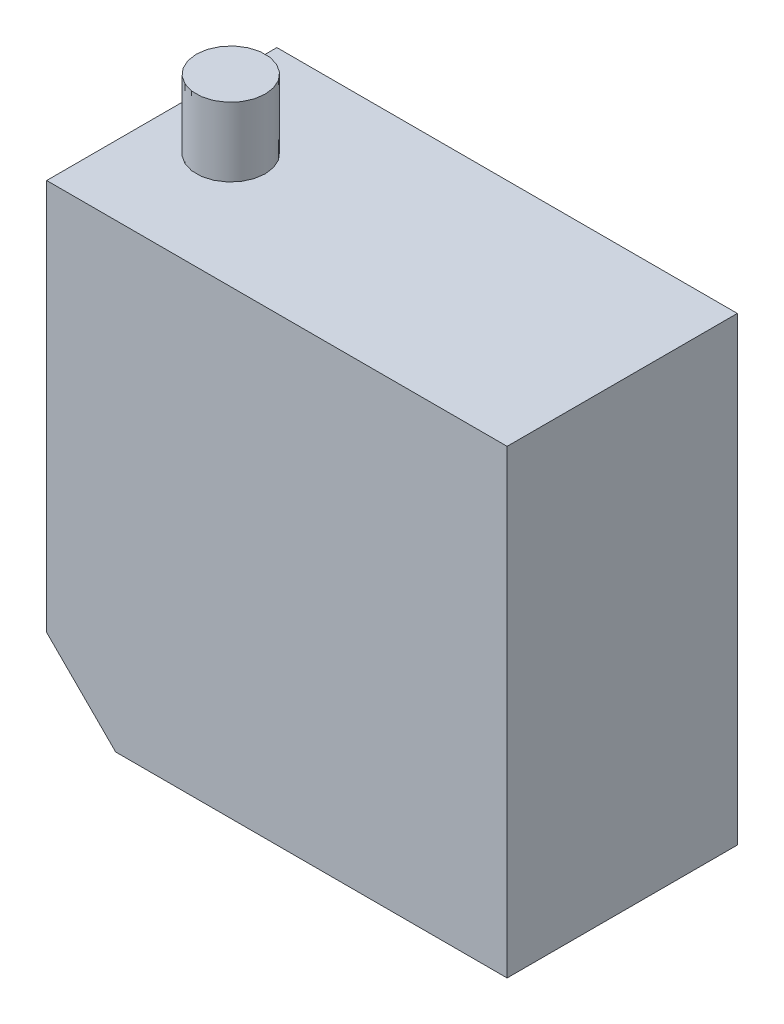
# Autodesk Inventor part: Finger Servo
Saved by Autodesk Inventor 2023 (Build 270158000, 158)
## iProperties
Created: 2023-09-27
Part Number: Finger Servo
Material: Generic
Document SubType Name: Modeling
Designer: Turnt
Density: 1 g/cm^3
Appearance: Default
Author: Turnt
Autodesk Inventor part; units mm, degrees
ref_plane "YZ Plane" through (0, 0, 0) normal (1, 0, 0) x (0, 1, 0)
ref_plane "XZ Plane" through (0, 0, 0) normal (0, 1, 0) x (-1, 0, 0)
ref_plane "XY Plane" through (0, 0, 0) normal (0, 0, 1) x (1, 0, 0)
sketch "Sketch1" plane through (0, 0, 0) normal (0, 0, 1) x (1, 0, 0)
  line L0 (3.8073, 0) -> (25.4, 0)
  line L1 (25.4, 0) -> (25.4, 25.4)
  line L2 (25.4, 25.4) -> (0, 25.4)
  line L3 (0, 25.4) -> (0, 3.8073)
  line L4 (0, 3.8073) -> (3.8073, 0)
  line L5 (0, 3.8073) -> (5.3843, 3.8073) construction
  point P0 (0, 0)
  dimension "d2" = 25.4
  dimension "d3" = 25.4
  dimension "d4" = 45
  constraints: 12 end point, 2 horizontal, 2 parallel, 1 equal length, 1 perpendicular
  measures "d2" distance of L2.end L1.end
  measures "d3" distance of L1.end L0.end
  measures "d4" angle of L4 L5
extrude "Extrusion1" add sketch "Sketch1" along normal blind 12.7
sketch "Sketch2" plane through (0, 25.4, 0) normal (0, 1, 0) x (1, 0, 0)
  line L0 (25.4, 0) -> (0, 0) projected
  line L1 (0, 0) -> (0, -12.7) projected
  line L2 (25.4, -12.7) -> (0, -12.7) projected
  line L3 (25.4, 0) -> (25.4, -12.7) projected
  line L4 (3.8073, 0) -> (3.8073, -12.7) projected
  circle A0 centre (3.8073, -6.35) radius 1.905
  dimension "d7" = 3.81
  constraints: 1 centre point, 1 midpoint
  measures "d7" diameter of A0
extrude "Extrusion2" add sketch "Sketch2" along normal blind 3.81 contours A0 L4 | L4 A0
body "Solid1"
